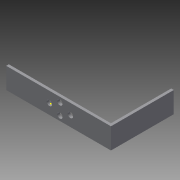
# Autodesk Inventor part: lBracketForLiftingBar
Saved by Autodesk Inventor 2015 (Build 190159000, 159)
## iProperties
Created: 2015-02-04
Part Number: lBracketForLiftingBar
Material: Generic
Document SubType Name: Modeling
Designer: Kingbob26
Density: 1 g/cm^3
Appearance: Default
Author: Kingbob26
Autodesk Inventor part; units mm, degrees
ref_plane "YZ Plane" through (0, 0, 0) normal (1, 0, 0) x (0, 1, 0)
ref_plane "XZ Plane" through (0, 0, 0) normal (0, 1, 0) x (-1, 0, 0)
ref_plane "XY Plane" through (0, 0, 0) normal (0, 0, 1) x (1, 0, 0)
sketch "Sketch1" plane through (0, 0, 0) normal (0, 0, 1) x (1, 0, 0)
  line L0 (57.15, 12.7) -> (-57.15, 12.7)
  line L1 (-57.15, 12.7) -> (-57.15, -12.7)
  line L2 (-57.15, -12.7) -> (57.15, -12.7)
  line L3 (57.15, -12.7) -> (57.15, 12.7)
  point P0 (0, 0)
  dimension "d0" = 114.3
  dimension "d1" = 25.4
  constraints: 8 end point, 2 parallel, 1 horizontal, 1 perpendicular
  measures "d0" distance of L2.end L1.end
  measures "d1" distance of L1.end L0.end
extrude "Extrusion1" add sketch "Sketch1" against normal blind 3.175
sketch "Sketch2" plane through (-57.15, -12.7, 0) normal (-1, 0, 0) x (0, 0, 1)
  line L0 (0, 25.4) -> (0, 0) projected
  line L1 (0, 25.4) -> (-3.175, 25.4) projected
  line L2 (-3.175, 0) -> (-3.175, 25.4) projected
  line L3 (0, 0) -> (-3.175, 0) projected
  point P0 (0, 12.7)
extrude "Extrusion2" cut sketch "Sketch2" against normal blind 3.175
sketch "Sketch4" plane through (0, 0, 0) normal (0, 0, 1) x (1, 0, 0)
  point P0 (0, 0)
sketch "Sketch5" plane through (0, 0, 0) normal (0, 0, 1) x (1, 0, 0)
  point P0 (0, 0)
sketch "Sketch6" plane through (57.15, -12.7, 0) normal (1, 0, 0) x (0, 0, -1)
  line L0 (0, 0) -> (0, 25.4) projected
  line L1 (0, 0) -> (3.175, 0) projected
  line L2 (3.175, 25.4) -> (3.175, 0) projected
  line L3 (0, 25.4) -> (3.175, 25.4) projected
  point P0 (0, 12.7)
extrude "Extrusion4" add sketch "Sketch6" along normal blind 12.7
sketch "Sketch7" plane through (0, 0, 0) normal (0, 0, 1) x (1, 0, 0)
  circle A0 centre (11.0998, -6.9088) radius 3.2639
  point P0 (0, 0)
  dimension "d11" = 6.5278
  constraints: 1 centre point
  measures "d11" diameter of A0
extrude "Extrusion5" cut sketch "Sketch7" against normal blind 12.7
sketch "Sketch8" plane through (0, 0, 0) normal (0, 0, 1) x (1, 0, 0)
  circle A0 centre (23.7998, 0) radius 3.2639
  point P0 (0, 0)
  dimension "d14" = 6.5278
  constraints: 1 centre point
  measures "d14" diameter of A0
extrude "Extrusion6" cut sketch "Sketch8" against normal blind 12.7
sketch "Sketch9" plane through (0, 0, 0) normal (0, 0, 1) x (1, 0, 0)
  circle A0 centre (11.0998, 6.9088) radius 3.2639
  point P0 (0, 0)
  dimension "d17" = 6.5278
  constraints: 1 centre point
  measures "d17" diameter of A0
extrude "Extrusion7" cut sketch "Sketch9" against normal blind 12.7
sketch "Sketch10" plane through (0, 0, 0) normal (0, 0, 1) x (1, 0, 0)
  circle A0 centre (-1.6002, 0) radius 3.2639
  point P0 (0, 0)
  dimension "d20" = 6.5278
  constraints: 1 centre point
  measures "d20" diameter of A0
extrude "Extrusion8" cut sketch "Sketch10" against normal blind 12.7
sketch "Sketch11" plane through (0, 0, 0) normal (0, 0, 1) x (1, 0, 0)
  line L0 (69.85, 12.7) -> (73.025, 12.7)
  line L1 (73.025, 12.7) -> (73.025, -12.7)
  line L2 (73.025, -12.7) -> (69.85, -12.7)
  line L3 (69.85, -12.7) -> (69.85, 12.7)
  point P0 (0, 0)
  dimension "d23" = 3.175
  constraints: 8 end point, 2 parallel, 1 horizontal, 1 perpendicular
  measures "d23" distance of L1.end L2.end
extrude "Extrusion9" add sketch "Sketch11" against normal blind 76.2
body "Solid1"
